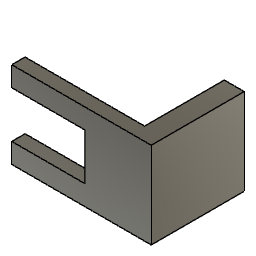
ppp2 v2 (Autodesk Fusion 360 design; units mm, degrees)
Autodesk Fusion 360 part; units mm, degrees
sketch "Sketch1" plane through (0, 0, 0) normal (0, 1, 0) x (1, 0, 0)
  line L0 (0, 0) -> (20, 0)
  line L1 (20, 0) -> (20, 13)
  line L2 (20, 13) -> (0, 13)
  line L3 (0, 3) -> (11, 3)
  line L4 (11, 3) -> (11, 10)
  line L5 (11, 10) -> (0, 10)
  line L6 (0, 13) -> (0, 10)
  line L7 (0, 3) -> (0, 0)
  circle A0 centre (15.5354, 6.5333) radius 3
  dimension "d2" = 6
  constraint horizontal L0
  constraint vertical L1
  constraint horizontal L2
  constraint vertical L6
  constraint coincident L0.start L7.end
  constraint horizontal L3
  constraint vertical L4
  constraint horizontal L5
  constraint coincident L3.start L6
  constraint collinear L6 L7
  measures "d2" diameter of A0
sketch "Sketch2" plane through (0, 0, 0) normal (0, 1, 0) x (-1, 0, 0)
  line L0 (0, -3) -> (-11, -3)
  line L1 (-20, -13) -> (0, -13)
  circle A0 centre (-15.5354, -6.5333) radius 3
  dimension "d3" = 11
  dimension "d4" = 20
  dimension "d5" = 6
  measures "d3" distance of L0.start L0.end
  measures "d4" distance of L1.start L1.end
  measures "d5" diameter of A0
extrude "Extrude1" add sketch "Sketch2" against normal blind 22
extrude "Extrude2" add sketch "Sketch1" against normal blind 2
sketch "Sketch3" plane through (20, 0, 0) normal (1, 0, 0) x (0, 1, 0)
  line L0 (0, -13) -> (0, 0)
  line L1 (0, 0) -> (-2, 0)
  line L2 (-2, 0) -> (-2, -13)
  line L3 (-2, -13) -> (0, -13)
extrude "Extrude3" add 1 faces at (15.9008, -22, -5.6024) along direction (0, -1, 0) blind 10
delete_face "DeleteFace1" 1 faces at (12.5503, -12, -6.2346)
extrude "Extrude4" add sketch "Sketch3" along normal blind 1
sketch "Sketch4" plane through (0, 0, 0) normal (0, 1, 0) x (1, 0, 0)
  line L0 (21, 0) -> (18, 0)
  line L1 (18, 0) -> (18, 13)
  line L2 (18, 13) -> (21, 13)
  line L3 (21, 13) -> (21, 0)
  dimension "d14" = 3
  dimension "d15" = 13
  constraint horizontal L0
  constraint vertical L1
  constraint horizontal L2
  constraint vertical L3
  measures "d14" distance of L0.start L0.end
  measures "d15" distance of L0.start L2.end
extrude "Extrude5" add sketch "Sketch4" along normal blind 10
extrude "Extrude6" add 1 faces at (19, 10, -4.3333) along direction (0, 1, 0) blind 2
